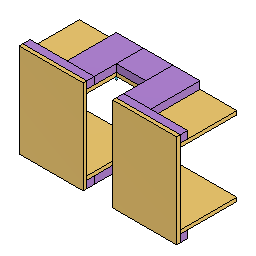
Hay Bale Chainsaw Notch Cutting Station A6 (Autodesk Fusion 360 design; units mm, degrees)
Autodesk Fusion 360 part; units mm, degrees
note: some values were not read from the file. Chosen so that the rebuilt part matches the saved one: which bodies a step acts on; which face or edge a step refers to. Set by a fixed rule: which sketch regions a step uses.
(part 1 of 2)
sketch "Sketch1" plane through (0, 0, 0) normal (0, 0, 1) x (1, 0, 0) in component "Large Box"
  line L0 (717.55, -273.05) -> (-717.55, -273.05)
  line L1 (-717.55, -273.05) -> (-717.55, 273.05)
  line L2 (-717.55, 273.05) -> (717.55, 273.05)
  line L3 (717.55, 273.05) -> (717.55, -273.05)
  line L4 (717.55, -273.05) -> (-717.55, 273.05) construction
  line L5 (-717.55, -273.05) -> (717.55, 273.05) construction
  line L6 (-717.55, -254) -> (717.55, -254)
  line L7 (-679.45, 254) -> (-679.45, -254)
  line L8 (-660.4, 254) -> (-660.4, -254)
  line L9 (679.45, 254) -> (679.45, -254)
  line L10 (679.45, 215.9) -> (717.55, 215.9)
  line L11 (679.45, -215.9) -> (717.55, -215.9)
  line L12 (-679.45, 215.9) -> (-717.55, 215.9)
  line L13 (-679.45, -215.9) -> (-717.55, -215.9)
  line L14 (660.4, 254) -> (660.4, -254)
  line L15 (114.3, -273.05) -> (114.3, -82.55)
  line L16 (114.3, -82.55) -> (266.7, -82.55)
  line L17 (266.7, -82.55) -> (266.7, -273.05)
  line L18 (114.3, -234.95) -> (-266.7, -234.95)
  line L19 (-266.7, -234.95) -> (-266.7, -254)
  line L20 (-285.75, -254) -> (-285.75, -234.95)
  line L21 (-285.75, -234.95) -> (-304.8, -234.95)
  line L22 (-304.8, -234.95) -> (-304.8, -254)
  line L23 (-323.85, -254) -> (-323.85, -234.95)
  line L24 (-323.85, -234.95) -> (-342.9, -234.95)
  line L25 (-342.9, -234.95) -> (-342.9, -254)
  line L26 (-533.4, -234.95) -> (-533.4, -254)
  line L27 (-514.35, -254) -> (-514.35, -234.95)
  line L28 (-609.6, -234.95) -> (-609.6, -254)
  line L29 (-590.55, -234.95) -> (-609.6, -234.95)
  line L30 (-628.65, -234.95) -> (-647.7, -234.95)
  line L31 (-571.5, -234.95) -> (-571.5, -254)
  line L32 (-628.65, -254) -> (-628.65, -234.95)
  line L33 (-514.35, -234.95) -> (-533.4, -234.95)
  line L34 (-552.45, -254) -> (-552.45, -234.95)
  line L35 (-590.55, -254) -> (-590.55, -234.95)
  line L36 (-552.45, -234.95) -> (-571.5, -234.95)
  line L37 (-647.7, -234.95) -> (-647.7, -254)
  line L38 (285.75, -234.95) -> (285.75, -254)
  line L39 (304.8, -254) -> (304.8, -234.95)
  line L40 (419.1, -234.95) -> (400.05, -234.95)
  line L41 (304.8, -234.95) -> (285.75, -234.95)
  line L42 (381, -234.95) -> (361.95, -234.95)
  line L43 (361.95, -234.95) -> (361.95, -254)
  line L44 (381, -254) -> (381, -234.95)
  line L45 (342.9, -254) -> (342.9, -234.95)
  line L46 (323.85, -234.95) -> (323.85, -254)
  line L47 (419.1, -254) -> (419.1, -234.95)
  line L48 (342.9, -234.95) -> (323.85, -234.95)
  line L49 (400.05, -234.95) -> (400.05, -254)
  line L50 (571.4775, -254) -> (571.4775, -234.95)
  line L51 (457.1775, -234.95) -> (438.1275, -234.95)
  line L52 (495.2775, -254) -> (495.2775, -234.95)
  line L53 (476.2275, -234.95) -> (476.2275, -254)
  line L54 (457.1775, -254) -> (457.1775, -234.95)
  line L55 (495.2775, -234.95) -> (476.2275, -234.95)
  line L56 (571.4775, -234.95) -> (552.4275, -234.95)
  line L57 (552.4275, -234.95) -> (552.4275, -254)
  line L58 (438.1275, -234.95) -> (438.1275, -254)
  line L59 (533.3775, -254) -> (533.3775, -234.95)
  line L60 (514.3275, -234.95) -> (514.3275, -254)
  line L61 (533.3775, -234.95) -> (514.3275, -234.95)
  line L62 (609.5775, -234.95) -> (590.5275, -234.95)
  line L63 (647.6775, -254) -> (647.6775, -234.95)
  line L64 (628.6275, -234.95) -> (628.6275, -254)
  line L65 (609.5775, -254) -> (609.5775, -234.95)
  line L66 (647.6775, -234.95) -> (628.6275, -234.95)
  line L67 (590.5275, -234.95) -> (590.5275, -254)
  line L68 (-400.05, 234.95) -> (-419.1, 234.95)
  line L69 (266.7, 234.95) -> (-266.7, 234.95)
  line L70 (628.6275, 234.95) -> (628.6275, 254)
  line L71 (381, 254) -> (381, 234.95)
  line L72 (342.9, 254) -> (342.9, 234.95)
  line L73 (609.5775, 234.95) -> (590.5275, 234.95)
  line L74 (419.1, 254) -> (419.1, 234.95)
  line L75 (647.6775, 234.95) -> (628.6275, 234.95)
  line L76 (-717.55, 254) -> (717.55, 254)
  line L77 (571.4775, 234.95) -> (552.4275, 234.95)
  line L78 (-514.35, 234.95) -> (-533.4, 234.95)
  line L79 (304.8, 234.95) -> (285.75, 234.95)
  line L80 (-285.75, 254) -> (-285.75, 234.95)
  line L81 (-361.95, 234.95) -> (-381, 234.95)
  line L82 (476.2275, 234.95) -> (476.2275, 254)
  line L83 (514.3275, 234.95) -> (514.3275, 254)
  line L84 (571.4775, 254) -> (571.4775, 234.95)
  line L85 (361.95, 234.95) -> (361.95, 254)
  line L86 (-381, 234.95) -> (-381, 254)
  line L87 (419.1, 234.95) -> (400.05, 234.95)
  line L88 (323.85, 234.95) -> (323.85, 254)
  line L89 (-590.55, 234.95) -> (-609.6, 234.95)
  line L90 (495.2775, 234.95) -> (476.2275, 234.95)
  line L91 (552.4275, 234.95) -> (552.4275, 254)
  line L92 (-438.15, 234.95) -> (-457.2, 234.95)
  line L93 (-514.35, 254) -> (-514.35, 234.95)
  line L94 (-533.4, 234.95) -> (-533.4, 254)
  line L95 (533.3775, 234.95) -> (514.3275, 234.95)
  line L96 (-609.6, 234.95) -> (-609.6, 254)
  line L97 (495.2775, 254) -> (495.2775, 234.95)
  line L98 (-400.05, 254) -> (-400.05, 234.95)
  line L99 (-552.45, 254) -> (-552.45, 234.95)
  line L100 (533.3775, 254) -> (533.3775, 234.95)
  line L101 (590.5275, 234.95) -> (590.5275, 254)
  line L102 (438.1275, 234.95) -> (438.1275, 254)
  line L103 (-419.1, 234.95) -> (-419.1, 254)
  line L104 (342.9, 234.95) -> (323.85, 234.95)
  line L105 (-628.65, 234.95) -> (-647.7, 234.95)
  line L106 (-285.75, 234.95) -> (-304.8, 234.95)
  line L107 (-266.7, 234.95) -> (-266.7, 254)
  line L108 (-323.85, 254) -> (-323.85, 234.95)
  line L109 (-590.55, 254) -> (-590.55, 234.95)
  line L110 (457.1775, 254) -> (457.1775, 234.95)
  line L111 (609.5775, 254) -> (609.5775, 234.95)
  line L112 (304.8, 254) -> (304.8, 234.95)
  line L113 (-342.9, 234.95) -> (-342.9, 254)
  line L114 (-571.5, 234.95) -> (-571.5, 254)
  line L115 (647.6775, 254) -> (647.6775, 234.95)
  line L116 (-323.85, 234.95) -> (-342.9, 234.95)
  line L117 (-552.45, 234.95) -> (-571.5, 234.95)
  line L118 (285.75, 234.95) -> (285.75, 254)
  line L119 (-361.95, 254) -> (-361.95, 234.95)
  line L120 (-304.8, 234.95) -> (-304.8, 254)
  line L121 (400.05, 234.95) -> (400.05, 254)
  line L122 (381, 234.95) -> (361.95, 234.95)
  line L123 (-628.65, 254) -> (-628.65, 234.95)
  line L124 (457.1775, 234.95) -> (438.1275, 234.95)
  line L125 (-476.25, 234.95) -> (-495.3, 234.95)
  line L126 (-476.25, 254) -> (-476.25, 234.95)
  line L127 (-647.7, 234.95) -> (-647.7, 254)
  line L128 (-438.15, 254) -> (-438.15, 234.95)
  line L129 (-495.3, 234.95) -> (-495.3, 254)
  line L130 (-457.2, 234.95) -> (-457.2, 254)
  line L131 (266.7, 234.95) -> (266.7, 254)
  line L132 (-361.95, -254) -> (-361.95, -234.95)
  line L133 (-438.15, -234.95) -> (-457.2, -234.95)
  line L134 (-361.95, -234.95) -> (-381, -234.95)
  line L135 (-400.05, -254) -> (-400.05, -234.95)
  line L136 (-457.2, -234.95) -> (-457.2, -254)
  line L137 (-381, -234.95) -> (-381, -254)
  line L138 (-400.05, -234.95) -> (-419.1, -234.95)
  line L139 (-438.15, -254) -> (-438.15, -234.95)
  line L140 (-419.1, -234.95) -> (-419.1, -254)
  line L141 (419.1, -234.95) -> (419.1, 234.95)
  line L142 (438.1275, 234.95) -> (438.1275, -234.95)
  line L143 (-495.3, -254) -> (-495.3, -234.95)
  line L144 (-495.3, -234.95) -> (-476.25, -234.95)
  line L145 (-476.25, -234.95) -> (-476.25, -254)
  line L146 (-514.35, 234.95) -> (-514.35, -234.95)
  line L147 (-495.3, -234.95) -> (-495.3, 234.95)
  circle A0 centre (88.9, -57.15) radius 4.7625
  circle A1 centre (292.1, -57.15) radius 4.7625
  line L148 (647.6775, 234.95) -> (628.6275, 234.95)
  line L149 (342.9, 234.95) -> (323.85, 234.95)
  line L150 (628.6275, 234.95) -> (628.6275, 254)
  line L151 (533.3775, 254) -> (533.3775, 234.95)
  line L152 (342.9, 254) -> (342.9, 234.95)
  line L153 (285.75, 234.95) -> (285.75, 254)
  line L154 (495.2775, 234.95) -> (476.2275, 234.95)
  line L155 (266.7, 234.95) -> (-266.7, 234.95)
  line L156 (419.1, 234.95) -> (400.05, 234.95)
  line L157 (476.2275, 234.95) -> (476.2275, 254)
  line L158 (114.3, -82.55) -> (266.7, -82.55)
  line L159 (304.8, 234.95) -> (285.75, 234.95)
  line L160 (419.1, 254) -> (419.1, 234.95)
  line L161 (438.1275, 234.95) -> (438.1275, 254)
  line L162 (571.4775, 254) -> (571.4775, 234.95)
  line L163 (609.5775, 234.95) -> (590.5275, 234.95)
  line L164 (381, 254) -> (381, 234.95)
  line L165 (-717.55, 273.05) -> (717.55, 273.05)
  line L166 (609.5775, 254) -> (609.5775, 234.95)
  line L167 (590.5275, 234.95) -> (590.5275, 254)
  line L168 (647.6775, 254) -> (647.6775, 234.95)
  line L169 (495.2775, 254) -> (495.2775, 234.95)
  line L170 (-717.55, -254) -> (717.55, -254)
  line L171 (514.3275, 234.95) -> (514.3275, 254)
  line L172 (323.85, 234.95) -> (323.85, 254)
  line L173 (679.45, 215.9) -> (717.55, 215.9)
  line L174 (457.1775, 234.95) -> (438.1275, 234.95)
  line L175 (304.8, 254) -> (304.8, 234.95)
  line L176 (457.1775, 254) -> (457.1775, 234.95)
  line L177 (717.55, -273.05) -> (-717.55, 273.05) construction
  line L178 (-717.55, -273.05) -> (717.55, 273.05) construction
  line L179 (571.4775, 234.95) -> (552.4275, 234.95)
  line L180 (342.9, -254) -> (342.9, -234.95)
  line L181 (-285.75, -254) -> (-285.75, -234.95)
  line L182 (-323.85, 234.95) -> (-342.9, 234.95)
  line L183 (266.7, 234.95) -> (266.7, 254)
  line L184 (381, 234.95) -> (361.95, 234.95)
  line L185 (-717.55, 254) -> (717.55, 254)
  line L186 (660.4, 254) -> (660.4, -254)
  line L187 (-660.4, 254) -> (-660.4, -254)
  line L188 (-514.35, 234.95) -> (-514.35, -234.95)
  line L189 (361.95, 234.95) -> (361.95, 254)
  line L190 (533.3775, 234.95) -> (514.3275, 234.95)
  line L191 (717.55, -273.05) -> (-717.55, -273.05)
  line L192 (419.1, -234.95) -> (419.1, 234.95)
  line L193 (717.55, 273.05) -> (717.55, -273.05)
  line L194 (-679.45, 254) -> (-679.45, -254)
  line L195 (-304.8, 234.95) -> (-304.8, 254)
  line L196 (552.4275, 234.95) -> (552.4275, 254)
  line L197 (400.05, 234.95) -> (400.05, 254)
  line L198 (679.45, 254) -> (679.45, -254)
  line L199 (-717.55, -273.05) -> (-717.55, 273.05)
  circle A2 centre (88.9, -57.15) radius 4.7625
  line L200 (438.1275, 234.95) -> (438.1275, -234.95)
  line L201 (-361.95, -234.95) -> (-381, -234.95)
  line L202 (114.3, -234.95) -> (-266.7, -234.95)
  line L203 (-342.9, 234.95) -> (-342.9, 254)
  line L204 (361.95, -234.95) -> (361.95, -254)
  line L205 (-342.9, -234.95) -> (-342.9, -254)
  line L206 (-514.35, 234.95) -> (-533.4, 234.95)
  line L207 (514.3275, -234.95) -> (514.3275, -254)
  line L208 (-266.7, 234.95) -> (-266.7, 254)
  line L209 (-476.25, 254) -> (-476.25, 234.95)
  line L210 (647.6775, -234.95) -> (628.6275, -234.95)
  line L211 (-647.7, -234.95) -> (-647.7, -254)
  line L212 (-552.45, 234.95) -> (-571.5, 234.95)
  line L213 (552.4275, -234.95) -> (552.4275, -254)
  line L214 (-514.35, 254) -> (-514.35, 234.95)
  line L215 (-590.55, 254) -> (-590.55, 234.95)
  line L216 (-476.25, -234.95) -> (-476.25, -254)
  line L217 (-381, -234.95) -> (-381, -254)
  line L218 (-323.85, -234.95) -> (-342.9, -234.95)
  line L219 (-495.3, -234.95) -> (-495.3, 234.95)
  line L220 (-285.75, -234.95) -> (-304.8, -234.95)
  line L221 (419.1, -254) -> (419.1, -234.95)
  line L222 (533.3775, -254) -> (533.3775, -234.95)
  line L223 (-323.85, 254) -> (-323.85, 234.95)
  line L224 (-495.3, 234.95) -> (-495.3, 254)
  line L225 (-590.55, 234.95) -> (-609.6, 234.95)
  line L226 (-476.25, 234.95) -> (-495.3, 234.95)
  line L227 (-361.95, 234.95) -> (-381, 234.95)
  line L228 (-571.5, 234.95) -> (-571.5, 254)
  line L229 (-285.75, 234.95) -> (-304.8, 234.95)
  line L230 (647.6775, -254) -> (647.6775, -234.95)
  line L231 (-514.35, -234.95) -> (-533.4, -234.95)
  line L232 (-400.05, 254) -> (-400.05, 234.95)
  line L233 (-628.65, -254) -> (-628.65, -234.95)
  line L234 (-419.1, 234.95) -> (-419.1, 254)
  line L235 (-304.8, -234.95) -> (-304.8, -254)
  line L236 (-533.4, 234.95) -> (-533.4, 254)
  line L237 (-609.6, -234.95) -> (-609.6, -254)
  line L238 (-679.45, 215.9) -> (-717.55, 215.9)
  line L239 (-400.05, -254) -> (-400.05, -234.95)
  line L240 (-457.2, 234.95) -> (-457.2, 254)
  line L241 (-361.95, 254) -> (-361.95, 234.95)
  line L242 (590.5275, -234.95) -> (590.5275, -254)
  line L243 (400.05, -234.95) -> (400.05, -254)
  line L244 (-552.45, 254) -> (-552.45, 234.95)
  line L245 (-361.95, -254) -> (-361.95, -234.95)
  line L246 (-323.85, -254) -> (-323.85, -234.95)
  line L247 (457.1775, -254) -> (457.1775, -234.95)
  line L248 (-400.05, -234.95) -> (-419.1, -234.95)
  line L249 (-381, 234.95) -> (-381, 254)
  line L250 (628.6275, -234.95) -> (628.6275, -254)
  line L251 (323.85, -234.95) -> (323.85, -254)
  line L252 (-266.7, -234.95) -> (-266.7, -254)
  line L253 (495.2775, -254) -> (495.2775, -234.95)
  line L254 (-514.35, -254) -> (-514.35, -234.95)
  line L255 (-285.75, 254) -> (-285.75, 234.95)
  line L256 (114.3, -273.05) -> (114.3, -82.55)
  line L257 (-438.15, 234.95) -> (-457.2, 234.95)
  line L258 (-679.45, -215.9) -> (-717.55, -215.9)
  line L259 (476.2275, -234.95) -> (476.2275, -254)
  line L260 (381, -254) -> (381, -234.95)
  line L261 (-628.65, 254) -> (-628.65, 234.95)
  line L262 (-590.55, -254) -> (-590.55, -234.95)
  line L263 (-628.65, -234.95) -> (-647.7, -234.95)
  line L264 (495.2775, -234.95) -> (476.2275, -234.95)
  line L265 (438.1275, -234.95) -> (438.1275, -254)
  line L266 (304.8, -254) -> (304.8, -234.95)
  line L267 (-495.3, -254) -> (-495.3, -234.95)
  line L268 (-609.6, 234.95) -> (-609.6, 254)
  line L269 (419.1, -234.95) -> (400.05, -234.95)
  line L270 (-438.15, -254) -> (-438.15, -234.95)
  line L271 (-552.45, -254) -> (-552.45, -234.95)
  line L272 (609.5775, -234.95) -> (590.5275, -234.95)
  line L273 (457.1775, -234.95) -> (438.1275, -234.95)
  line L274 (679.45, -215.9) -> (717.55, -215.9)
  line L275 (-628.65, 234.95) -> (-647.7, 234.95)
  line L276 (304.8, -234.95) -> (285.75, -234.95)
  line L277 (-590.55, -234.95) -> (-609.6, -234.95)
  line L278 (-419.1, -234.95) -> (-419.1, -254)
  line L279 (285.75, -234.95) -> (285.75, -254)
  line L280 (-457.2, -234.95) -> (-457.2, -254)
  line L281 (533.3775, -234.95) -> (514.3275, -234.95)
  line L282 (-533.4, -234.95) -> (-533.4, -254)
  line L283 (-438.15, -234.95) -> (-457.2, -234.95)
  line L284 (-495.3, -234.95) -> (-476.25, -234.95)
  line L285 (609.5775, -254) -> (609.5775, -234.95)
  line L286 (-438.15, 254) -> (-438.15, 234.95)
  line L287 (-647.7, 234.95) -> (-647.7, 254)
  line L288 (-571.5, -234.95) -> (-571.5, -254)
  circle A3 centre (292.1, -57.15) radius 4.7625
  line L289 (266.7, -82.55) -> (266.7, -273.05)
  line L290 (-552.45, -234.95) -> (-571.5, -234.95)
  line L291 (571.4775, -234.95) -> (552.4275, -234.95)
  line L292 (381, -234.95) -> (361.95, -234.95)
  line L293 (-400.05, 234.95) -> (-419.1, 234.95)
  line L294 (342.9, -234.95) -> (323.85, -234.95)
  line L295 (571.4775, -254) -> (571.4775, -234.95)
  line L296 (647.6775, 234.95) -> (628.6275, 234.95)
  line L297 (342.9, 234.95) -> (323.85, 234.95)
  line L298 (628.6275, 234.95) -> (628.6275, 254)
  line L299 (533.3775, 254) -> (533.3775, 234.95)
  line L300 (342.9, 254) -> (342.9, 234.95)
  line L301 (285.75, 234.95) -> (285.75, 254)
  line L302 (495.2775, 234.95) -> (476.2275, 234.95)
  line L303 (266.7, 234.95) -> (-266.7, 234.95)
  line L304 (419.1, 234.95) -> (400.05, 234.95)
  line L305 (476.2275, 234.95) -> (476.2275, 254)
  line L306 (114.3, -82.55) -> (266.7, -82.55)
  line L307 (304.8, 234.95) -> (285.75, 234.95)
  line L308 (419.1, 254) -> (419.1, 234.95)
  line L309 (438.1275, 234.95) -> (438.1275, 254)
  line L310 (571.4775, 254) -> (571.4775, 234.95)
  line L311 (609.5775, 234.95) -> (590.5275, 234.95)
  line L312 (381, 254) -> (381, 234.95)
  line L313 (-717.55, 273.05) -> (717.55, 273.05)
  line L314 (609.5775, 254) -> (609.5775, 234.95)
  line L315 (590.5275, 234.95) -> (590.5275, 254)
  line L316 (647.6775, 254) -> (647.6775, 234.95)
  line L317 (495.2775, 254) -> (495.2775, 234.95)
  line L318 (-717.55, -254) -> (717.55, -254)
  line L319 (514.3275, 234.95) -> (514.3275, 254)
  line L320 (323.85, 234.95) -> (323.85, 254)
  line L321 (679.45, 215.9) -> (717.55, 215.9)
  line L322 (457.1775, 234.95) -> (438.1275, 234.95)
  line L323 (304.8, 254) -> (304.8, 234.95)
  line L324 (457.1775, 254) -> (457.1775, 234.95)
  line L325 (717.55, -273.05) -> (-717.55, 273.05) construction
  line L326 (-717.55, -273.05) -> (717.55, 273.05) construction
  line L327 (571.4775, 234.95) -> (552.4275, 234.95)
  line L328 (342.9, -254) -> (342.9, -234.95)
  line L329 (-285.75, -254) -> (-285.75, -234.95)
  line L330 (-323.85, 234.95) -> (-342.9, 234.95)
  line L331 (266.7, 234.95) -> (266.7, 254)
  line L332 (381, 234.95) -> (361.95, 234.95)
  line L333 (-717.55, 254) -> (717.55, 254)
  line L334 (660.4, 254) -> (660.4, -254)
  line L335 (-660.4, 254) -> (-660.4, -254)
  line L336 (-514.35, 234.95) -> (-514.35, -234.95)
  line L337 (361.95, 234.95) -> (361.95, 254)
  line L338 (533.3775, 234.95) -> (514.3275, 234.95)
  line L339 (717.55, -273.05) -> (-717.55, -273.05)
  line L340 (419.1, -234.95) -> (419.1, 234.95)
  line L341 (717.55, 273.05) -> (717.55, -273.05)
  line L342 (-679.45, 254) -> (-679.45, -254)
  line L343 (-304.8, 234.95) -> (-304.8, 254)
  line L344 (552.4275, 234.95) -> (552.4275, 254)
  line L345 (400.05, 234.95) -> (400.05, 254)
  line L346 (679.45, 254) -> (679.45, -254)
  line L347 (-717.55, -273.05) -> (-717.55, 273.05)
  circle A4 centre (88.9, -57.15) radius 4.7625
  line L348 (438.1275, 234.95) -> (438.1275, -234.95)
  line L349 (-361.95, -234.95) -> (-381, -234.95)
  line L350 (114.3, -234.95) -> (-266.7, -234.95)
  line L351 (-342.9, 234.95) -> (-342.9, 254)
  line L352 (361.95, -234.95) -> (361.95, -254)
  line L353 (-342.9, -234.95) -> (-342.9, -254)
  line L354 (-514.35, 234.95) -> (-533.4, 234.95)
  line L355 (514.3275, -234.95) -> (514.3275, -254)
  line L356 (-266.7, 234.95) -> (-266.7, 254)
  line L357 (-476.25, 254) -> (-476.25, 234.95)
  line L358 (647.6775, -234.95) -> (628.6275, -234.95)
  line L359 (-647.7, -234.95) -> (-647.7, -254)
  line L360 (-552.45, 234.95) -> (-571.5, 234.95)
  line L361 (552.4275, -234.95) -> (552.4275, -254)
  line L362 (-514.35, 254) -> (-514.35, 234.95)
  line L363 (-590.55, 254) -> (-590.55, 234.95)
  line L364 (-476.25, -234.95) -> (-476.25, -254)
  line L365 (-381, -234.95) -> (-381, -254)
  line L366 (-323.85, -234.95) -> (-342.9, -234.95)
  line L367 (-495.3, -234.95) -> (-495.3, 234.95)
  line L368 (-285.75, -234.95) -> (-304.8, -234.95)
  line L369 (419.1, -254) -> (419.1, -234.95)
  line L370 (533.3775, -254) -> (533.3775, -234.95)
  line L371 (-323.85, 254) -> (-323.85, 234.95)
  line L372 (-495.3, 234.95) -> (-495.3, 254)
  line L373 (-590.55, 234.95) -> (-609.6, 234.95)
  line L374 (-476.25, 234.95) -> (-495.3, 234.95)
  line L375 (-361.95, 234.95) -> (-381, 234.95)
  line L376 (-571.5, 234.95) -> (-571.5, 254)
  line L377 (-285.75, 234.95) -> (-304.8, 234.95)
  line L378 (647.6775, -254) -> (647.6775, -234.95)
  line L379 (-514.35, -234.95) -> (-533.4, -234.95)
  line L380 (-400.05, 254) -> (-400.05, 234.95)
  line L381 (-628.65, -254) -> (-628.65, -234.95)
  line L382 (-419.1, 234.95) -> (-419.1, 254)
  line L383 (-304.8, -234.95) -> (-304.8, -254)
  line L384 (-533.4, 234.95) -> (-533.4, 254)
  line L385 (-609.6, -234.95) -> (-609.6, -254)
  line L386 (-679.45, 215.9) -> (-717.55, 215.9)
  line L387 (-400.05, -254) -> (-400.05, -234.95)
  line L388 (-457.2, 234.95) -> (-457.2, 254)
  line L389 (-361.95, 254) -> (-361.95, 234.95)
  line L390 (590.5275, -234.95) -> (590.5275, -254)
  line L391 (400.05, -234.95) -> (400.05, -254)
  line L392 (-552.45, 254) -> (-552.45, 234.95)
  line L393 (-361.95, -254) -> (-361.95, -234.95)
  line L394 (-323.85, -254) -> (-323.85, -234.95)
  line L395 (457.1775, -254) -> (457.1775, -234.95)
  line L396 (-400.05, -234.95) -> (-419.1, -234.95)
  line L397 (-381, 234.95) -> (-381, 254)
  line L398 (628.6275, -234.95) -> (628.6275, -254)
  line L399 (323.85, -234.95) -> (323.85, -254)
  line L400 (-266.7, -234.95) -> (-266.7, -254)
  line L401 (495.2775, -254) -> (495.2775, -234.95)
  line L402 (-514.35, -254) -> (-514.35, -234.95)
  line L403 (-285.75, 254) -> (-285.75, 234.95)
  line L404 (114.3, -273.05) -> (114.3, -82.55)
  line L405 (-438.15, 234.95) -> (-457.2, 234.95)
  line L406 (-679.45, -215.9) -> (-717.55, -215.9)
  line L407 (476.2275, -234.95) -> (476.2275, -254)
  line L408 (381, -254) -> (381, -234.95)
  line L409 (-628.65, 254) -> (-628.65, 234.95)
  line L410 (-590.55, -254) -> (-590.55, -234.95)
  line L411 (-628.65, -234.95) -> (-647.7, -234.95)
  line L412 (495.2775, -234.95) -> (476.2275, -234.95)
  line L413 (438.1275, -234.95) -> (438.1275, -254)
  line L414 (304.8, -254) -> (304.8, -234.95)
  line L415 (-495.3, -254) -> (-495.3, -234.95)
  line L416 (-609.6, 234.95) -> (-609.6, 254)
  line L417 (419.1, -234.95) -> (400.05, -234.95)
  line L418 (-438.15, -254) -> (-438.15, -234.95)
  line L419 (-552.45, -254) -> (-552.45, -234.95)
  line L420 (609.5775, -234.95) -> (590.5275, -234.95)
  line L421 (457.1775, -234.95) -> (438.1275, -234.95)
  line L422 (679.45, -215.9) -> (717.55, -215.9)
  line L423 (-628.65, 234.95) -> (-647.7, 234.95)
  line L424 (304.8, -234.95) -> (285.75, -234.95)
  line L425 (-590.55, -234.95) -> (-609.6, -234.95)
  line L426 (-419.1, -234.95) -> (-419.1, -254)
  line L427 (285.75, -234.95) -> (285.75, -254)
  line L428 (-457.2, -234.95) -> (-457.2, -254)
  line L429 (533.3775, -234.95) -> (514.3275, -234.95)
  line L430 (-533.4, -234.95) -> (-533.4, -254)
  line L431 (-438.15, -234.95) -> (-457.2, -234.95)
  line L432 (-495.3, -234.95) -> (-476.25, -234.95)
  line L433 (609.5775, -254) -> (609.5775, -234.95)
  line L434 (-438.15, 254) -> (-438.15, 234.95)
  line L435 (-647.7, 234.95) -> (-647.7, 254)
  line L436 (-571.5, -234.95) -> (-571.5, -254)
  circle A5 centre (292.1, -57.15) radius 4.7625
  line L437 (266.7, -82.55) -> (266.7, -273.05)
  line L438 (-552.45, -234.95) -> (-571.5, -234.95)
  line L439 (571.4775, -234.95) -> (552.4275, -234.95)
  line L440 (381, -234.95) -> (361.95, -234.95)
  line L441 (-400.05, 234.95) -> (-419.1, 234.95)
  line L442 (342.9, -234.95) -> (323.85, -234.95)
  line L443 (571.4775, -254) -> (571.4775, -234.95)
  point P0 (190.5, -82.55)
  point P1 (190.5, -82.55)
  point P2 (190.5, -82.55)
  dimension "d1" = 546.1
  dimension "d2" = 1435.1
  dimension "d4" = 38.1
  dimension "d5" = 19.05
  dimension "d7" = 19.05
  dimension "d8" = 38.1
  dimension "d11" = 19.05
  dimension "d12" = 190.5
  dimension "d13" = 152.4
  dimension "d14" = 927.1
  dimension "d15" = 19.05
  dimension "d17" = 19.05
  dimension "d18" = 19.05
  dimension "d19" = 19.05
  dimension "d24" = 19.05
  dimension "d25" = 19.05
  dimension "d26" = 19.05
  dimension "d27" = 19.05
  dimension "d33" = 927.1
  dimension "d37" = 19.05
  dimension "d38" = 19.05
  dimension "d39" = 19.05
  dimension "d40" = 19.05
  dimension "d41" = 19.05
  dimension "d42" = 19.05
  dimension "d45" = 19.05
  dimension "d46" = 19.05
  dimension "d47" = 19.0275
  dimension "d48" = 19.05
  dimension "d50" = 19.05
  dimension "d51" = 19.05
  dimension "d52" = 19.05
  dimension "d53" = 19.05
  dimension "d54" = 19.05
  dimension "d55" = 19.05
  dimension "d56" = 19.05
  dimension "d57" = 19.05
  dimension "d58" = 19.05
  dimension "d59" = 19.05
  dimension "d60" = 19.05
  dimension "d61" = 19.05
  dimension "d64" = 19.05
  dimension "d68" = 19.05
  dimension "d69" = 19.05
  dimension "d70" = 19.05
  dimension "d71" = 19.05
  dimension "d72" = 19.05
  dimension "d73" = 19.05
  dimension "d76" = 19.05
  dimension "d77" = 19.0275
  dimension "d78" = 19.05
  dimension "d81" = 19.05
  dimension "d82" = 19.05
  dimension "d99" = 19.05
  dimension "d100" = 38.1
  dimension "d102" = 469.9
  dimension "d103" = 1320.8
  dimension "d104" = 19.05
  dimension "d105" = 19.05
  dimension "d106" = 19.05
  dimension "d128" = 9.525
  dimension "d129" = 25.4
  dimension "d130" = 25.4
  dimension "d131" = 9.525
  dimension "d132" = 25.4
  dimension "d139" = 546.1
  dimension "d140" = 1435.1
  dimension "d141" = 38.1
  dimension "d142" = 19.05
  dimension "d143" = 19.05
  dimension "d144" = 38.1
  dimension "d145" = 19.05
  dimension "d146" = 190.5
  dimension "d147" = 152.4
  dimension "d148" = 927.1
  dimension "d149" = 19.05
  dimension "d150" = 19.05
  dimension "d151" = 19.05
  dimension "d152" = 19.05
  dimension "d153" = 19.05
  dimension "d154" = 19.05
  dimension "d155" = 19.05
  dimension "d156" = 19.05
  dimension "d157" = 927.1
  dimension "d158" = 19.05
  dimension "d159" = 19.05
  dimension "d160" = 19.05
  dimension "d161" = 19.05
  dimension "d162" = 19.05
  dimension "d163" = 19.05
  dimension "d164" = 19.05
  dimension "d165" = 19.05
  dimension "d166" = 19.0275
  dimension "d167" = 19.05
  dimension "d168" = 19.05
  dimension "d169" = 19.05
  dimension "d170" = 19.05
  dimension "d171" = 19.05
  dimension "d172" = 19.05
  dimension "d173" = 19.05
  dimension "d174" = 19.05
  dimension "d175" = 19.05
  dimension "d176" = 19.05
  dimension "d177" = 19.05
  dimension "d178" = 19.05
  dimension "d179" = 19.05
  dimension "d180" = 19.05
  dimension "d181" = 19.05
  dimension "d182" = 19.05
  dimension "d183" = 19.05
  dimension "d184" = 19.05
  dimension "d185" = 19.05
  dimension "d186" = 19.05
  dimension "d187" = 19.05
  dimension "d188" = 19.0275
  dimension "d189" = 19.05
  dimension "d190" = 19.05
  dimension "d191" = 19.05
  dimension "d192" = 19.05
  dimension "d193" = 38.1
  dimension "d194" = 469.9
  dimension "d195" = 1320.8
  dimension "d196" = 19.05
  dimension "d197" = 19.05
  dimension "d198" = 19.05
  dimension "d199" = 9.525
  dimension "d200" = 25.4
  dimension "d201" = 25.4
  dimension "d202" = 9.525
  dimension "d203" = 25.4
  dimension "d204" = 546.1
  dimension "d205" = 1435.1
  dimension "d206" = 38.1
  dimension "d207" = 19.05
  dimension "d208" = 19.05
  dimension "d209" = 38.1
  dimension "d210" = 19.05
  dimension "d211" = 190.5
  dimension "d212" = 152.4
  dimension "d213" = 927.1
  dimension "d214" = 19.05
  dimension "d215" = 19.05
  dimension "d216" = 19.05
  dimension "d217" = 19.05
  dimension "d218" = 19.05
  dimension "d219" = 19.05
  dimension "d220" = 19.05
  dimension "d221" = 19.05
  dimension "d222" = 927.1
  dimension "d223" = 19.05
  dimension "d224" = 19.05
  dimension "d225" = 19.05
  dimension "d226" = 19.05
  dimension "d227" = 19.05
  dimension "d228" = 19.05
  dimension "d229" = 19.05
  dimension "d230" = 19.05
  dimension "d231" = 19.0275
  dimension "d232" = 19.05
  dimension "d233" = 19.05
  dimension "d234" = 19.05
  dimension "d235" = 19.05
  dimension "d236" = 19.05
  dimension "d237" = 19.05
  dimension "d238" = 19.05
  dimension "d239" = 19.05
  dimension "d240" = 19.05
  dimension "d241" = 19.05
  dimension "d242" = 19.05
  dimension "d243" = 19.05
  dimension "d244" = 19.05
  dimension "d245" = 19.05
  dimension "d246" = 19.05
  dimension "d247" = 19.05
  dimension "d248" = 19.05
  dimension "d249" = 19.05
  dimension "d250" = 19.05
  dimension "d251" = 19.05
  dimension "d252" = 19.05
  dimension "d253" = 19.0275
  dimension "d254" = 19.05
  dimension "d255" = 19.05
  dimension "d256" = 19.05
  dimension "d257" = 19.05
  dimension "d258" = 38.1
  dimension "d259" = 469.9
  dimension "d260" = 1320.8
  dimension "d261" = 19.05
  dimension "d262" = 19.05
  dimension "d263" = 19.05
  dimension "d264" = 9.525
  dimension "d265" = 25.4
  dimension "d266" = 25.4
  dimension "d267" = 9.525
  dimension "d268" = 25.4
  constraint horizontal L0
  constraint perpendicular L0 L1
  constraint parallel L0 L2
  constraint parallel L1 L3
  constraint coincident L4 origin
  constraint coincident L5 origin
  constraint coincident L1 L6.start
  constraint coincident L3 L6.end
  constraint perpendicular L3 L6
  constraint coincident L6 L7.end
  constraint coincident L6 L8.end
  constraint perpendicular L6 L8
  constraint coincident L6 L9.end
  constraint perpendicular L6 L9
  constraint coincident L9 L10.start
  constraint coincident L3 L10.end
  constraint perpendicular L3 L10
  constraint coincident L9 L11.start
  constraint coincident L3 L11.end
  constraint perpendicular L3 L11
  constraint coincident L7 L12.start
  constraint coincident L1 L12.end
  constraint perpendicular L1 L12
  constraint coincident L7 L13.start
  constraint coincident L1 L13.end
  constraint perpendicular L1 L13
  constraint collinear L11 L13
  constraint collinear L10 L12
  constraint equal L11 L13
  constraint coincident L6 L14.end
  constraint coincident L0 L15.start
  constraint perpendicular L0 L15
  constraint perpendicular L15 L16
  constraint coincident L0 L17.end
  constraint perpendicular L0 L17
  constraint coincident L15 L18.start
  constraint perpendicular L15 L18
  constraint coincident L6 L19.end
  constraint perpendicular L6 L19
  constraint coincident L6 L20.start
  constraint perpendicular L6 L20
  constraint perpendicular L15 L21
  constraint coincident L6 L22.end
  constraint perpendicular L6 L22
  constraint collinear L18 L21
  constraint coincident L6 L23.start
  constraint perpendicular L6 L23
  constraint perpendicular L23 L24
  constraint coincident L6 L25.end
  constraint perpendicular L6 L25
  constraint equal L22 L23
  constraint equal L21 L24
  constraint perpendicular L34 L36
  constraint perpendicular L29 L31
  constraint perpendicular L30 L31
  constraint equal L26 L34
  constraint equal L26 L35
  constraint equal L26 L32
  constraint equal L33 L36
  constraint equal L29 L33
  constraint equal L30 L33
  constraint coincident L6 L27.start
  constraint coincident L6 L26.end
  constraint coincident L6 L34.start
  constraint coincident L6 L31.end
  constraint coincident L6 L35.start
  constraint coincident L6 L28.end
  constraint coincident L6 L32.start
  constraint coincident L6 L37.end
  constraint collinear L21 L33
  constraint vertical L27
  constraint vertical L34
  constraint vertical L35
  constraint vertical L32
  constraint midpoint L16 P2
  constraint horizontal L41
  constraint vertical L38
  constraint vertical L39
  constraint horizontal L48
  constraint vertical L45
  constraint horizontal L42
  constraint horizontal L40
  constraint coincident L6 L38.end
  constraint coincident L6 L39.start
  constraint coincident L6 L46.end
  constraint coincident L6 L45.start
  constraint coincident L6 L43.end
  constraint coincident L6 L44.start
  constraint coincident L6 L49.end
  constraint coincident L6 L47.start
  constraint collinear L21 L41
  constraint collinear L41 L48
  constraint collinear L42 L48
  constraint collinear L40 L42
  constraint horizontal L51
  constraint vertical L58
  constraint vertical L54
  constraint horizontal L55
  constraint vertical L52
  constraint horizontal L61
  constraint horizontal L56
  constraint collinear L51 L55
  constraint collinear L55 L61
  constraint collinear L56 L61
  constraint horizontal L62
  constraint vertical L67
  constraint vertical L65
  constraint horizontal L66
  constraint vertical L63
  constraint collinear L62 L66
  constraint equal L21 L41
  constraint equal L41 L48
  constraint equal L42 L48
  constraint equal L40 L42
  constraint equal L40 L51
  constraint equal L51 L55
  constraint equal L55 L61
  constraint equal L56 L61
  constraint equal L56 L62
  constraint equal L62 L66
  constraint coincident L6 L63.start
  constraint coincident L6 L64.end
  constraint coincident L6 L65.start
  constraint coincident L6 L67.end
  constraint coincident L6 L50.start
  constraint coincident L6 L57.end
  constraint coincident L6 L59.start
  constraint coincident L6 L60.end
  constraint coincident L6 L52.start
  constraint coincident L6 L53.end
  constraint coincident L6 L54.start
  constraint collinear L56 L62
  constraint collinear L40 L51
  constraint vertical L47
  constraint vertical L49
  constraint vertical L59
  constraint coincident L107.end L76
  constraint perpendicular L76 L107
  constraint coincident L80.start L76
  constraint perpendicular L76 L80
  constraint coincident L120.end L76
  constraint perpendicular L76 L120
  constraint collinear L69 L106
  constraint coincident L108.start L76
  constraint perpendicular L76 L108
  constraint perpendicular L108 L116
  constraint coincident L113.end L76
  constraint perpendicular L76 L113
  constraint coincident L119.start L76
  constraint perpendicular L76 L119
  constraint perpendicular L81 L113
  constraint coincident L86.end L76
  constraint perpendicular L76 L86
  constraint coincident L98.start L76
  constraint perpendicular L76 L98
  constraint perpendicular L68 L113
  constraint coincident L103.end L76
  constraint perpendicular L76 L103
  constraint coincident L128.start L76
  constraint perpendicular L76 L128
  constraint perpendicular L92 L113
  constraint coincident L130.end L76
  constraint perpendicular L76 L130
  constraint coincident L126.start L76
  constraint perpendicular L76 L126
  constraint perpendicular L113 L125
  constraint coincident L129.end L76
  constraint perpendicular L76 L129
  constraint equal L108 L120
  constraint equal L119 L120
  constraint equal L98 L120
  constraint equal L120 L128
  constraint equal L120 L126
  constraint equal L106 L116
  constraint equal L81 L106
  constraint equal L68 L106
  constraint equal L92 L106
  constraint equal L106 L125
  constraint perpendicular L99 L117
  constraint perpendicular L89 L114
  constraint perpendicular L105 L114
  constraint equal L94 L99
  constraint equal L94 L109
  constraint equal L94 L123
  constraint equal L78 L117
  constraint equal L78 L89
  constraint equal L78 L105
  constraint coincident L93.start L76
  constraint coincident L94.end L76
  constraint coincident L99.start L76
  constraint coincident L114.end L76
  constraint coincident L109.start L76
  constraint coincident L96.end L76
  constraint coincident L123.start L76
  constraint coincident L127.end L76
  constraint collinear L78 L106
  constraint coincident L118.end L76
  constraint coincident L112.start L76
  constraint coincident L88.end L76
  constraint coincident L72.start L76
  constraint coincident L85.end L76
  constraint coincident L71.start L76
  constraint coincident L121.end L76
  constraint coincident L74.start L76
  constraint collinear L79 L106
  constraint collinear L79 L104
  constraint collinear L104 L122
  constraint collinear L87 L122
  constraint collinear L90 L124
  constraint collinear L90 L95
  constraint collinear L77 L95
  constraint collinear L73 L75
  constraint equal L79 L106
  constraint equal L79 L104
  constraint equal L104 L122
  constraint equal L87 L122
  constraint equal L87 L124
  constraint equal L90 L124
  constraint equal L90 L95
  constraint equal L77 L95
  constraint equal L73 L77
  constraint equal L73 L75
  constraint coincident L115.start L76
  constraint coincident L70.end L76
  constraint coincident L111.start L76
  constraint coincident L101.end L76
  constraint coincident L84.start L76
  constraint coincident L91.end L76
  constraint coincident L100.start L76
  constraint coincident L83.end L76
  constraint coincident L97.start L76
  constraint coincident L82.end L76
  constraint coincident L110.start L76
  constraint collinear L73 L77
  constraint collinear L87 L124
  constraint horizontal L76
  constraint coincident L1 L76.start
  constraint coincident L7.start L76
  constraint coincident L8.start L76
  constraint coincident L3 L76.end
  constraint coincident L9.start L76
  constraint coincident L14.start L76
  constraint coincident L76 L131.end
  constraint perpendicular L76 L131
  constraint collinear L17 L131
  constraint collinear L19 L107
  constraint vertical L94
  constraint vertical L114
  constraint vertical L96
  constraint vertical L127
  constraint vertical L118
  constraint vertical L112
  constraint vertical L72
  constraint vertical L71
  constraint vertical L74
  constraint vertical L110
  constraint vertical L97
  constraint vertical L100
  constraint vertical L111
  constraint vertical L84
  constraint vertical L115
  constraint coincident L102.end L76
  constraint collinear L38 L118
  constraint perpendicular L132 L134
  constraint perpendicular L137 L138
  constraint perpendicular L133 L137
  constraint vertical L132
  constraint vertical L135
  constraint vertical L139
  constraint vertical L136
  constraint coincident L6 L136.end
  constraint coincident L6 L139.start
  constraint coincident L6 L140.end
  constraint coincident L6 L135.start
  constraint coincident L6 L137.end
  constraint coincident L6 L132.start
  constraint coincident L6 L58.end
  constraint coincident L6 L143.start
  constraint perpendicular L6 L143
  constraint perpendicular L143 L144
  constraint coincident L6 L145.end
  constraint perpendicular L6 L145
  constraint collinear L33 L144
  constraint equal L33 L144
  constraint equal L136 L145
  constraint equal L136 L140
  constraint equal L137 L140
  constraint equal L133 L144
  constraint equal L133 L138
  constraint vertical L37
  constraint coincident L114.start L117.end
  constraint perpendicular L33 L146
  constraint horizontal A0.centre A1.centre
  constraint horizontal L191
  constraint perpendicular L191 L199
  constraint parallel L165 L191
  constraint parallel L193 L199
  constraint coincident origin L177
  constraint coincident origin L178
  constraint coincident L6.start L199
  constraint coincident L6.end L193
  constraint perpendicular L170 L193
  constraint coincident L7.end L170
  constraint coincident L8.end L170
  constraint perpendicular L170 L187
  constraint coincident L9.end L170
  constraint perpendicular L170 L198
  constraint coincident L10.start L198
  constraint coincident L10.end L193
  constraint perpendicular L173 L193
  constraint coincident L11.start L198
  constraint coincident L11.end L193
  constraint perpendicular L193 L274
  constraint coincident L12.start L194
  constraint coincident L12.end L199
  constraint perpendicular L199 L238
  constraint coincident L13.start L194
  constraint coincident L13.end L199
  constraint perpendicular L199 L258
  constraint collinear L258 L274
  constraint collinear L173 L238
  constraint equal L258 L274
  constraint coincident L14.end L170
  constraint coincident L15.start L191
  constraint perpendicular L191 L256
  constraint perpendicular L158 L256
  constraint coincident L17.end L191
  constraint perpendicular L191 L289
  constraint coincident L18.start L256
  constraint perpendicular L202 L256
  constraint coincident L19.end L170
  constraint perpendicular L170 L252
  constraint coincident L20.start L170
  constraint perpendicular L170 L181
  constraint perpendicular L220 L256
  constraint coincident L22.end L170
  constraint perpendicular L170 L235
  constraint collinear L202 L220
  constraint coincident L23.start L170
  constraint perpendicular L170 L246
  constraint perpendicular L218 L246
  constraint coincident L25.end L170
  constraint perpendicular L170 L205
  constraint equal L235 L246
  constraint equal L218 L220
  constraint perpendicular L271 L290
  constraint perpendicular L277 L288
  constraint perpendicular L263 L288
  constraint equal L271 L282
  constraint equal L262 L282
  constraint equal L233 L282
  constraint equal L231 L290
  constraint equal L231 L277
  constraint equal L231 L263
  constraint coincident L27.start L170
  constraint coincident L26.end L170
  constraint coincident L34.start L170
  constraint coincident L31.end L170
  constraint coincident L35.start L170
  constraint coincident L28.end L170
  constraint coincident L32.start L170
  constraint coincident L37.end L170
  constraint collinear L220 L231
  constraint vertical L254
  constraint vertical L271
  constraint vertical L262
  constraint vertical L233
  constraint midpoint P2 L158
  constraint horizontal L276
  constraint vertical L279
  constraint vertical L266
  constraint horizontal L294
  constraint vertical L180
  constraint horizontal L292
  constraint horizontal L269
  constraint coincident L38.end L170
  constraint coincident L39.start L170
  constraint coincident L46.end L170
  constraint coincident L45.start L170
  constraint coincident L43.end L170
  constraint coincident L44.start L170
  constraint coincident L49.end L170
  constraint coincident L47.start L170
  constraint collinear L220 L276
  constraint collinear L276 L294
  constraint collinear L292 L294
  constraint collinear L269 L292
  constraint horizontal L273
  constraint vertical L265
  constraint vertical L247
  constraint horizontal L264
  constraint vertical L253
  constraint horizontal L281
  constraint horizontal L291
  constraint collinear L264 L273
  constraint collinear L264 L281
  constraint collinear L281 L291
  constraint horizontal L272
  constraint vertical L242
  constraint vertical L285
  constraint horizontal L210
  constraint vertical L230
  constraint collinear L210 L272
  constraint equal L220 L276
  constraint equal L276 L294
  constraint equal L292 L294
  constraint equal L269 L292
  constraint equal L269 L273
  constraint equal L264 L273
  constraint equal L264 L281
  constraint equal L281 L291
  constraint equal L272 L291
  constraint equal L210 L272
  constraint coincident L63.start L170
  constraint coincident L64.end L170
  constraint coincident L65.start L170
  constraint coincident L67.end L170
  constraint coincident L50.start L170
  constraint coincident L57.end L170
  constraint coincident L59.start L170
  constraint coincident L60.end L170
  constraint coincident L52.start L170
  constraint coincident L53.end L170
  constraint coincident L54.start L170
  constraint collinear L272 L291
  constraint collinear L269 L273
  constraint vertical L221
  constraint vertical L243
  constraint vertical L222
  constraint coincident L107.end L185
  constraint perpendicular L185 L208
  constraint coincident L80.start L185
  constraint perpendicular L185 L255
  constraint coincident L120.end L185
  constraint perpendicular L185 L195
  constraint collinear L155 L229
  constraint coincident L108.start L185
  constraint perpendicular L185 L223
  constraint perpendicular L182 L223
  constraint coincident L113.end L185
  constraint perpendicular L185 L203
  constraint coincident L119.start L185
  constraint perpendicular L185 L241
  constraint perpendicular L203 L227
  constraint coincident L86.end L185
  constraint perpendicular L185 L249
  constraint coincident L98.start L185
  constraint perpendicular L185 L232
  constraint perpendicular L203 L293
  constraint coincident L103.end L185
  constraint perpendicular L185 L234
  constraint coincident L128.start L185
  constraint perpendicular L185 L286
  constraint perpendicular L203 L257
  constraint coincident L130.end L185
  constraint perpendicular L185 L240
  constraint coincident L126.start L185
  constraint perpendicular L185 L209
  constraint perpendicular L203 L226
  constraint coincident L129.end L185
  constraint perpendicular L185 L224
  constraint equal L195 L223
  constraint equal L195 L241
  constraint equal L195 L232
  constraint equal L195 L286
  constraint equal L195 L209
  constraint equal L182 L229
  constraint equal L227 L229
  constraint equal L229 L293
  constraint equal L229 L257
  constraint equal L226 L229
  constraint perpendicular L212 L244
  constraint perpendicular L225 L228
  constraint perpendicular L228 L275
  constraint equal L236 L244
  constraint equal L215 L236
  constraint equal L236 L261
  constraint equal L206 L212
  constraint equal L206 L225
  constraint equal L206 L275
  constraint coincident L93.start L185
  constraint coincident L94.end L185
  constraint coincident L99.start L185
  constraint coincident L114.end L185
  constraint coincident L109.start L185
  constraint coincident L96.end L185
  constraint coincident L123.start L185
  constraint coincident L127.end L185
  constraint collinear L206 L229
  constraint coincident L118.end L185
  constraint coincident L112.start L185
  constraint coincident L88.end L185
  constraint coincident L72.start L185
  constraint coincident L85.end L185
  constraint coincident L71.start L185
  constraint coincident L121.end L185
  constraint coincident L74.start L185
  constraint collinear L159 L229
  constraint collinear L149 L159
  constraint collinear L149 L184
  constraint collinear L156 L184
  constraint collinear L154 L174
  constraint collinear L154 L190
  constraint collinear L179 L190
  constraint collinear L148 L163
  constraint equal L159 L229
  constraint equal L149 L159
  constraint equal L149 L184
  constraint equal L156 L184
  constraint equal L156 L174
  constraint equal L154 L174
  constraint equal L154 L190
  constraint equal L179 L190
  constraint equal L163 L179
  constraint equal L148 L163
  constraint coincident L115.start L185
  constraint coincident L70.end L185
  constraint coincident L111.start L185
  constraint coincident L101.end L185
  constraint coincident L84.start L185
  constraint coincident L91.end L185
  constraint coincident L100.start L185
  constraint coincident L83.end L185
  constraint coincident L97.start L185
  constraint coincident L82.end L185
  constraint coincident L110.start L185
  constraint collinear L163 L179
  constraint collinear L156 L174
  constraint horizontal L185
  constraint coincident L76.start L199
  constraint coincident L7.start L185
  constraint coincident L8.start L185
  constraint coincident L76.end L193
  constraint coincident L9.start L185
  constraint coincident L14.start L185
  constraint coincident L131.end L185
  constraint perpendicular L183 L185
  constraint collinear L183 L289
  constraint collinear L208 L252
  constraint vertical L236
  constraint vertical L228
  constraint vertical L268
  constraint vertical L287
  constraint vertical L153
  constraint vertical L175
  constraint vertical L152
  constraint vertical L164
  constraint vertical L160
  constraint vertical L176
  constraint vertical L169
  constraint vertical L151
  constraint vertical L166
  constraint vertical L162
  constraint vertical L168
  constraint coincident L102.end L185
  constraint collinear L153 L279
  constraint perpendicular L201 L245
  constraint perpendicular L217 L248
  constraint perpendicular L217 L283
  constraint vertical L245
  constraint vertical L239
  constraint vertical L270
  constraint vertical L280
  constraint coincident L136.end L170
  constraint coincident L139.start L170
  constraint coincident L140.end L170
  constraint coincident L135.start L170
  constraint coincident L137.end L170
  constraint coincident L132.start L170
  constraint coincident L58.end L170
  constraint coincident L143.start L170
  constraint perpendicular L170 L267
  constraint perpendicular L267 L284
  constraint coincident L145.end L170
  constraint perpendicular L170 L216
  constraint collinear L231 L284
  constraint equal L231 L284
  constraint equal L216 L280
  constraint equal L278 L280
  constraint equal L217 L278
  constraint equal L283 L284
  constraint equal L248 L283
  constraint vertical L211
  constraint perpendicular L188 L231
  constraint horizontal L339
  constraint perpendicular L339 L347
  constraint parallel L313 L339
  constraint parallel L341 L347
  constraint coincident origin L325
  constraint coincident origin L326
  constraint coincident L6.start L347
  constraint coincident L6.end L341
  constraint perpendicular L318 L341
  constraint coincident L7.end L318
  constraint coincident L8.end L318
  constraint perpendicular L318 L335
  constraint coincident L9.end L318
  constraint perpendicular L318 L346
  constraint coincident L10.start L346
  constraint coincident L10.end L341
  constraint perpendicular L321 L341
  constraint coincident L11.start L346
  constraint coincident L11.end L341
  constraint perpendicular L341 L422
  constraint coincident L12.start L342
  constraint coincident L12.end L347
  constraint perpendicular L347 L386
  constraint coincident L13.start L342
  constraint coincident L13.end L347
  constraint perpendicular L347 L406
  constraint collinear L406 L422
  constraint collinear L321 L386
  constraint equal L406 L422
  constraint coincident L14.end L318
  constraint coincident L15.start L339
  constraint perpendicular L339 L404
  constraint perpendicular L306 L404
  constraint coincident L17.end L339
  constraint perpendicular L339 L437
  constraint coincident L18.start L404
  constraint perpendicular L350 L404
  constraint coincident L19.end L318
  constraint perpendicular L318 L400
  constraint coincident L20.start L318
  constraint perpendicular L318 L329
  constraint perpendicular L368 L404
  constraint coincident L22.end L318
  constraint perpendicular L318 L383
  constraint collinear L350 L368
  constraint coincident L23.start L318
  constraint perpendicular L318 L394
  constraint perpendicular L366 L394
  constraint coincident L25.end L318
  constraint perpendicular L318 L353
  constraint equal L383 L394
  constraint equal L366 L368
  constraint perpendicular L419 L438
  constraint perpendicular L425 L436
  constraint perpendicular L411 L436
  constraint equal L419 L430
  constraint equal L410 L430
  constraint equal L381 L430
  constraint equal L379 L438
  constraint equal L379 L425
  constraint equal L379 L411
  constraint coincident L27.start L318
  constraint coincident L26.end L318
  constraint coincident L34.start L318
  constraint coincident L31.end L318
  constraint coincident L35.start L318
  constraint coincident L28.end L318
  constraint coincident L32.start L318